Autodesk Fusion 360 part; units mm, degrees
(part 6 of 6)
  spline S46 degree 5 poles (13.4255, 19.2781) (13.4314, 19.2865) (13.4429, 19.3035) (13.4596, 19.3295) (13.4806, 19.3648) (13.5051, 19.41) (13.5284, 19.456) (13.551, 19.5024) (13.5732, 19.5491) (13.5951, 19.596) (13.6167, 19.6431) (13.6379, 19.6904) (13.6586, 19.7381) (13.6787, 19.786) (13.6983, 19.8343) (13.7172, 19.883) (13.7357, 19.9319) (13.7538, 19.9811) (13.7716, 20.0304) (13.789, 20.08) (13.8061, 20.1297) (13.8228, 20.1796) (13.8392, 20.2297) (13.8552, 20.28) (13.8708, 20.3305) (13.886, 20.3812) (13.9009, 20.4321) (13.9155, 20.4832) (13.9297, 20.5344) (13.9437, 20.5858) (13.9573, 20.6374) (13.9706, 20.6891) (13.9836, 20.7409) (13.9963, 20.793) (14.0087, 20.8451) (14.0208, 20.8974) (14.0326, 20.9499) (14.0441, 21.0025) (14.0553, 21.0552) (14.0663, 21.1081) (14.0769, 21.1611) (14.0873, 21.2142) (14.0974, 21.2675) (14.1072, 21.3208) (14.1167, 21.3743) (14.126, 21.428) (14.135, 21.4817) (14.1437, 21.5356) (14.1522, 21.5896) (14.1603, 21.6436) (14.1683, 21.6978) (14.1759, 21.7522) (14.1833, 21.8066) (14.1905, 21.8611) (14.1974, 21.9157) (14.204, 21.9705) (14.2104, 22.0253) (14.2165, 22.0802) (14.2224, 22.1353) (14.228, 22.1904) (14.2334, 22.2456) (14.2385, 22.301) (14.2434, 22.3564) (14.248, 22.4119) (14.2524, 22.4675) (14.2566, 22.5232) (14.2605, 22.5789) (14.2642, 22.6348) (14.2676, 22.6908) (14.2708, 22.7468) (14.2737, 22.8029) (14.2759, 22.8478) (14.2774, 22.8816) (14.2784, 22.9041) (14.2788, 22.9154) knots 0 0 0 0 0 0 0.01428571 0.02857143 0.04285714 0.05714286 0.07142857 0.08571429 0.1 0.11428571 0.12857143 0.14285714 0.15714286 0.17142857 0.18571429 0.2 0.21428571 0.22857143 0.24285714 0.25714286 0.27142857 0.28571429 0.3 0.31428571 0.32857143 0.34285714 0.35714286 0.37142857 0.38571429 0.4 0.41428571 0.42857143 0.44285714 0.45714286 0.47142857 0.48571429 0.5 0.51428571 0.52857143 0.54285714 0.55714286 0.57142857 0.58571429 0.6 0.61428571 0.62857143 0.64285714 0.65714286 0.67142857 0.68571429 0.7 0.71428571 0.72857143 0.74285714 0.75714286 0.77142857 0.78571429 0.8 0.81428571 0.82857143 0.84285714 0.85714286 0.87142857 0.88571429 0.9 0.91428571 0.92857143 0.94285714 0.95714286 0.97142857 0.98571429 1 1 1 1 1 1
  arc A100 (14.2788, 22.9154) -> (13.0373, 23.6438) centre (0, 0) ccw
  spline S47 degree 5 poles (13.0373, 23.6438) (13.0277, 23.6379) (13.0085, 23.6261) (12.9798, 23.6083) (12.9416, 23.5845) (12.894, 23.5545) (12.8467, 23.5244) (12.7995, 23.4941) (12.7525, 23.4637) (12.7058, 23.433) (12.6592, 23.4022) (12.6128, 23.3713) (12.5666, 23.3402) (12.5206, 23.3089) (12.4748, 23.2774) (12.4292, 23.2458) (12.3838, 23.2139) (12.3387, 23.182) (12.2937, 23.1498) (12.2489, 23.1175) (12.2044, 23.085) (12.1601, 23.0523) (12.116, 23.0195) (12.0721, 22.9865) (12.0284, 22.9533) (11.985, 22.9199) (11.9417, 22.8864) (11.8987, 22.8527) (11.856, 22.8188) (11.8135, 22.7847) (11.7712, 22.7505) (11.7291, 22.7161) (11.6873, 22.6815) (11.6457, 22.6467) (11.6044, 22.6117) (11.5633, 22.5766) (11.5225, 22.5412) (11.482, 22.5057) (11.4417, 22.47) (11.4016, 22.4341) (11.3619, 22.398) (11.3224, 22.3618) (11.2832, 22.3253) (11.2443, 22.2886) (11.2056, 22.2518) (11.1673, 22.2147) (11.1292, 22.1775) (11.0914, 22.1401) (11.054, 22.1024) (11.0168, 22.0646) (10.98, 22.0265) (10.9435, 21.9883) (10.9074, 21.9498) (10.8716, 21.911) (10.8362, 21.8721) (10.8011, 21.8329) (10.7664, 21.7935) (10.732, 21.754) (10.6979, 21.7142) (10.6642, 21.6742) (10.631, 21.6339) (10.5984, 21.5933) (10.5663, 21.5523) (10.5348, 21.511) (10.5039, 21.4694) (10.4733, 21.4275) (10.4431, 21.3856) (10.4131, 21.3434) (10.3836, 21.301) (10.3548, 21.2583) (10.3273, 21.2148) (10.3067, 21.1792) (10.2922, 21.1521) (10.283, 21.1337) (10.2785, 21.1244) knots -1 -1 -1 -1 -1 -1 -0.98571429 -0.97142857 -0.95714286 -0.94285714 -0.92857143 -0.91428571 -0.9 -0.88571429 -0.87142857 -0.85714286 -0.84285714 -0.82857143 -0.81428571 -0.8 -0.78571429 -0.77142857 -0.75714286 -0.74285714 -0.72857143 -0.71428571 -0.7 -0.68571429 -0.67142857 -0.65714286 -0.64285714 -0.62857143 -0.61428571 -0.6 -0.58571429 -0.57142857 -0.55714286 -0.54285714 -0.52857143 -0.51428571 -0.5 -0.48571429 -0.47142857 -0.45714286 -0.44285714 -0.42857143 -0.41428571 -0.4 -0.38571429 -0.37142857 -0.35714286 -0.34285714 -0.32857143 -0.31428571 -0.3 -0.28571429 -0.27142857 -0.25714286 -0.24285714 -0.22857143 -0.21428571 -0.2 -0.18571429 -0.17142857 -0.15714286 -0.14285714 -0.12857143 -0.11428571 -0.1 -0.08571429 -0.07142857 -0.05714286 -0.04285714 -0.02857143 -0.01428571 0 0 0 0 0 0
  line L49 (10.2785, 21.1244) -> (10.0602, 20.6767)
  arc A101 (9.4018, 20.4415) -> (10.0602, 20.6767) centre (9.6107, 20.8958) ccw
  circle A102 centre (0, 0) radius 22.5
  circle A103 centre (0, 0) radius 27
  line L50 (-38.7828, -16.9438) -> (0.0188, 0.0082) construction
  line L51 (0, 0) -> (20.6182, 9.0079) construction
  line L52 (11.8156, 24.2774) -> (0, 0) construction
  circle A104 centre (0.0188, 0.0082) radius 20
  circle A105 centre (0, 0) radius 5
  circle A106 centre (0, 0) radius 7.5
  dimension "d14" = 40
  dimension "d15" = 15
  dimension "d16" = 10
  constraint coincident A0.centre A2.centre
  constraint coincident A98.end A102
  constraint concentric A102 A103
  constraint coincident S46.end A103
  constraint coincident A1.centre A40.centre
  constraint midpoint A90 L51.end
  constraint coincident A103 L52.start
  constraint coincident L50.end A104.centre
  constraint concentric A103 A105
  constraint concentric A105 A106
  measures "d14" diameter of A104
  measures "d15" diameter of A106
  measures "d16" diameter of A105
extrude "Extruir9" add sketch "Boceto8" along normal blind 1 contours A2 A6 A10 A14 A18 A22 A26 A30 A34 A38 A42 A46 A50 A54 A58 A62 A66 A70 A74 A78 A82 A86 A90 A94 A98 A102 | A106
hole "Agujero1" at (0, 0, 0) direction (-1, 0, 0) diameter 3 depth 14 tip angle 180 counterbore diameter 5 counterbore depth 2
hole "Agujero2" at (0, -38.7828, -16.9438) direction (-1, 0, 0) diameter 3 depth 14 tip angle 180 counterbore diameter 5 counterbore depth 2
sketch "Boceto9" plane through (0, 0, 0) normal (1, 0, 0) x (0, 1, 0)
  circle A0 centre (0.0188, 0.0082) radius 20
  circle A1 centre (0, 0) radius 7.5
  circle A2 centre (0, 0) radius 11.1575
  dimension "d29" = 7
  text T0 "EPLA    ARI" font "Arial Black" height 7 bold align left spacing 1 along the path A2 letters at x, y, angle (-21.9304, 3.4662, 71.8674) (-15.6319, 15.7671, 35.6023) (-3.5374, 21.8772, 0.7226) (9.6637, 20.0414, -35.6161) (18.9054, 11.2132, -63.5812) (21.3346, 5.2901, -80.3284) (21.954, -1.0819, -97.0755) (20.7111, -7.362, -113.8227) (16.5569, -14.8632, -141.7878) (3.4432, -21.9816, 179.0292) (-9.4281, -19.8802, 149.6665)
  constraint concentric A1 A2
extrude "Extruir10" add sketch "Boceto9" along normal blind 1 text T0
equation "d30 = 'EPLA    ARI'"
named bodies: "Engranaje tracción"
